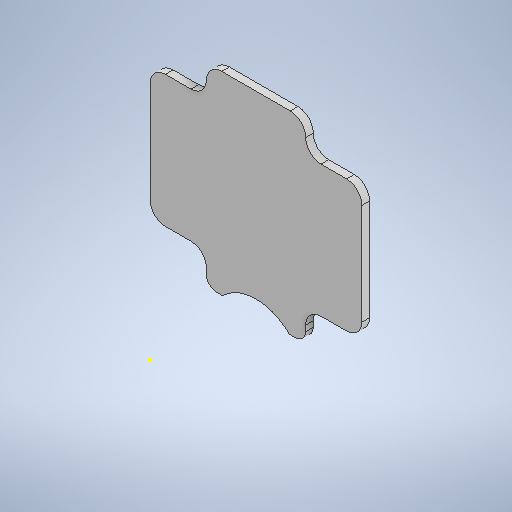
# Autodesk Inventor part: anchor-screen-cover
Saved by Autodesk Inventor 2025.2 (Build 292293000, 293)
## iProperties
Created: 2025-05-20
Part Number: anchor-screen-cover
Material: Generic
Document SubType Name: Modeling
Designer: tyson
Density: 1 g/cm^3
Appearance: Default
Autodesk Inventor part; units mm, degrees
ref_plane "YZ Plane" through (0, 0, 0) normal (1, 0, 0) x (0, 1, 0)
ref_plane "XZ Plane" through (0, 0, 0) normal (0, 1, 0) x (-1, 0, 0)
ref_plane "XY Plane" through (0, 0, 0) normal (0, 0, 1) x (1, 0, 0)
sketch "Sketch1" plane through (0, 0, 0) normal (0, 0, 1) x (1, 0, 0)
  point P0 (0, 0)
sketch "0" plane through (0, 0, 0) normal (0, 0, 1) x (1, 0, 0)
  arc A0 (31.9, 54.31) -> (34.9, 51.31) centre (34.9, 54.31) ccw
  line L0 (34.9, 51.31) -> (39.9, 51.31)
  arc A1 (42.9, 48.31) -> (39.9, 51.31) centre (39.9, 48.31) ccw
  line L1 (42.9, 48.31) -> (42.9, 28.56)
  arc A2 (39.9, 25.56) -> (42.9, 28.56) centre (39.9, 28.56) ccw
  line L2 (39.9, 25.56) -> (34.9, 25.56)
  line L3 (15.6769, 19.4231) -> (14.5, 19.4231)
  arc A3 (12.5, 21.4231) -> (14.5, 19.4231) centre (14.5, 21.4231) ccw
  line L4 (12.5, 21.4231) -> (12.5, 22.56)
  arc A4 (12.5, 22.56) -> (9.5, 25.56) centre (9.5, 22.56) ccw
  line L5 (9.5, 51.31) -> (4.5, 51.31)
  arc A5 (4.5, 51.31) -> (1.5, 48.31) centre (4.5, 48.31) ccw
  line L6 (1.5, 48.31) -> (1.5, 28.56)
  arc A6 (1.5, 28.56) -> (4.5, 25.56) centre (4.5, 28.56) ccw
  line L7 (4.5, 25.56) -> (9.5, 25.56)
  arc A7 (31.9, 54.31) -> (28.9, 57.31) centre (28.9, 54.31) ccw
  line L8 (28.9, 57.31) -> (15.5, 57.31)
  arc A8 (15.5, 57.31) -> (12.5, 54.31) centre (15.5, 54.31) ccw
  line L9 (28.7231, 19.4231) -> (29.9, 19.4231)
  arc A9 (29.9, 19.4231) -> (31.9, 21.4231) centre (29.9, 21.4231) ccw
  line L10 (31.9, 21.4231) -> (31.9, 22.56)
  line L11 (12.705, 53.275) -> (12.705, 23.375)
  line L12 (15.805, 56.275) -> (28.595, 56.275)
  line L13 (31.595, 53.275) -> (31.595, 23.375)
  line L14 (30.345, 22.125) -> (14.055, 22.125)
  circle A10 centre (9.5, 54.31) radius 2
  circle A11 centre (9.5, 22.56) radius 2
  circle A12 centre (34.9, 22.56) radius 2
  circle A13 centre (34.9, 54.31) radius 2
  circle A14 centre (9.5, 54.31) radius 3
  circle A15 centre (9.5, 22.56) radius 3
  circle A16 centre (34.9, 22.56) radius 3
  circle A17 centre (34.9, 54.31) radius 3
  circle A18 centre (22.2, 12.9) radius 8.75
  circle A19 centre (22.2, 12.9) radius 9.225
  arc A20 (28.7231, 19.4231) -> (15.6769, 19.4231) centre (22.2, 12.9) ccw
  line L15 (22.2, 12.9) -> (28.7231, 19.4231)
  line L16 (22.2, 12.9) -> (31.425, 12.9)
  line L17 (22.2, 12.9) -> (15.6769, 19.4231)
  arc A21 (9.5, 51.31) -> (12.5, 54.31) centre (9.5, 54.31) ccw
  arc A22 (34.9, 25.56) -> (31.9, 22.56) centre (34.9, 22.56) ccw
  point P0 (31.9, 54.31)
  point P1 (12.5, 54.31)
  point P2 (4.5, 51.31)
  point P3 (1.5, 48.31)
  constraints: 36 end point, 26 point on circle, 23 centre point
extrude "Extrusion1" add sketch "0" along normal blind 1.5 contours A0 L0 A1 L1 A2 L2 A16 L10 A9 L9 A19 L3 A3 L4 A4 L7 A6 L6 A5 L5 A14 A8 L8 A7
body "Solid1"
